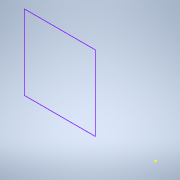
# Autodesk Inventor part: electronics box
Saved by Autodesk Inventor 2022 (Build 260153000, 153)
## iProperties
Created: 2022-02-07
Part Number: electronics box
Material: Generic
Document SubType Name: Modeling
Designer: efred
Density: 1 g/cm^3
Appearance: Default
Author: efred
Autodesk Inventor part; units mm, degrees
ref_plane "YZ Plane" through (0, 0, 0) normal (1, 0, 0) x (0, 1, 0)
ref_plane "XZ Plane" through (0, 0, 0) normal (0, 1, 0) x (-1, 0, 0)
ref_plane "XY Plane" through (0, 0, 0) normal (0, 0, 1) x (1, 0, 0)
sketch "Sketch1" plane through (0, 0, 0) normal (0, 0, 1) x (1, 0, 0)
  line L0 (-184.2713, 193.3742) -> (-404.2713, 193.3742)
  line L1 (-404.2713, 193.3742) -> (-404.2713, -23.6258)
  line L2 (-404.2713, -23.6258) -> (-184.2713, -23.6258)
  line L3 (-184.2713, -23.6258) -> (-184.2713, 193.3742)
  line L4 (-196.3213, 183.3742) -> (-190.7713, 183.3742) projected
  point P0 (0, 0)
  dimension "d2" = 10
  dimension "d3" = 217
  dimension "d4" = 220
  constraints: 8 end point, 2 parallel, 1 horizontal, 1 perpendicular
  measures "d2" distance between parallel lines of L4 L0
  measures "d3" distance of L2.end L0.start
  measures "d4" distance of L1.end L2.end
extrude "Extrusion1" add sketch "Sketch1" against normal blind 10
sketch "Sketch2" plane through (0, 0, -10) normal (0, 0, -1) x (-1, 0, 0)
  line L0 (404.2713, -23.6258) -> (404.2713, 193.3742) projected
  line L1 (404.2713, 193.3742) -> (184.2713, 193.3742) projected
  line L2 (184.2713, 193.3742) -> (184.2713, -23.6258) projected
  line L3 (184.2713, -23.6258) -> (404.2713, -23.6258) projected
  circle A0 centre (400.2713, 80.3742) radius 1.5 projected
  circle A1 centre (363.2713, 80.3742) radius 1.5 projected
  circle A2 centre (400.2713, 93.3742) radius 1.5 projected
  circle A3 centre (363.2713, 93.3742) radius 1.5 projected
  circle A4 centre (363.2713, 130.3742) radius 1.5 projected
  circle A5 centre (400.2713, 130.3742) radius 1.5 projected
  circle A6 centre (400.2713, 143.3742) radius 1.5 projected
  circle A7 centre (400.2713, 180.3742) radius 1.5 projected
  circle A8 centre (363.2713, 180.3742) radius 1.5 projected
  circle A9 centre (363.2713, 143.3742) radius 1.5 projected
  circle A10 centre (320.7713, 167.5022) radius 1.375 projected
  circle A11 centre (320.7713, 109.5022) radius 1.375 projected
  circle A12 centre (271.7713, 109.5022) radius 1.375 projected
  circle A13 centre (271.7713, 167.5022) radius 1.375 projected
  circle A14 centre (244.7713, 128.3904) radius 2 projected
  circle A15 centre (244.7713, 100.8904) radius 2 projected
  circle A16 centre (263.7713, 100.8904) radius 2 projected
  circle A17 centre (263.7713, 128.3904) radius 2 projected
  line L4 (264.4663, 47.3647) -> (264.4663, 46.7297) projected
  arc A18 (264.4663, 46.7297) -> (264.5298, 46.6662) centre (264.5298, 46.7297) ccw projected
  line L5 (264.5298, 46.6662) -> (266.003, 46.6662) projected
  arc A19 (266.0665, 46.6027) -> (266.003, 46.6662) centre (266.003, 46.6027) ccw projected
  line L6 (266.0665, 39.1097) -> (266.0665, 46.6027) projected
  arc A20 (266.003, 39.0462) -> (266.0665, 39.1097) centre (266.003, 39.1097) ccw projected
  line L7 (266.003, 39.0462) -> (264.5298, 39.0462) projected
  arc A21 (264.5298, 39.0462) -> (264.4663, 38.9827) centre (264.5298, 38.9827) ccw projected
  line L8 (264.4663, 38.9827) -> (264.4663, 38.3477) projected
  arc A22 (264.4028, 38.2842) -> (264.4663, 38.3477) centre (264.4028, 38.3477) ccw projected
  line L9 (253.6713, 38.2842) -> (264.4028, 38.2842) projected
  line L10 (253.6713, 35.9982) -> (253.6713, 38.2842) projected
  line L11 (253.6713, 35.9982) -> (255.1953, 34.4742) projected
  line L12 (351.7153, 34.4742) -> (255.1953, 34.4742) projected
  line L13 (351.7153, 34.4742) -> (355.2713, 38.0302) projected
  line L14 (355.2713, 72.6504) -> (355.2713, 38.0302) projected
  line L15 (352.7313, 75.1904) -> (355.2713, 72.6504) projected
  line L16 (352.7313, 86.127) -> (352.7313, 75.1904) projected
  line L17 (350.9679, 87.8904) -> (352.7313, 86.127) projected
  line L18 (255.1953, 87.8904) -> (350.9679, 87.8904) projected
  line L19 (255.1953, 87.8904) -> (253.6713, 86.3664) projected
  line L20 (253.6713, 78.6194) -> (253.6713, 86.3664) projected
  line L21 (260.6817, 78.6194) -> (253.6713, 78.6194) projected
  line L22 (260.6817, 78.6829) -> (260.6817, 78.6194) projected
  line L23 (263.6281, 78.6829) -> (260.6817, 78.6829) projected
  line L24 (263.6281, 66.6179) -> (263.6281, 78.6829) projected
  line L25 (263.6281, 66.6179) -> (260.6817, 66.6179) projected
  line L26 (260.6817, 66.6179) -> (260.6817, 66.6814) projected
  line L27 (253.6713, 66.6814) -> (260.6817, 66.6814) projected
  line L28 (253.6713, 47.4282) -> (253.6713, 66.6814) projected
  line L29 (264.4028, 47.4282) -> (253.6713, 47.4282) projected
  arc A23 (264.4663, 47.3647) -> (264.4028, 47.4282) centre (264.4028, 47.3647) ccw projected
  line L30 (301.2963, 35.8204) -> (301.2963, 38.2698) projected
  line L31 (285.5991, 35.8204) -> (301.2963, 35.8204) projected
  line L32 (285.5991, 38.2698) -> (285.5991, 35.8204) projected
  line L33 (301.2963, 38.2698) -> (285.5991, 38.2698) projected
  line L34 (274.9311, 84.1566) -> (295.6829, 84.1566) projected
  line L35 (274.9311, 86.6204) -> (274.9311, 84.1566) projected
  line L36 (295.6829, 86.6204) -> (274.9311, 86.6204) projected
  line L37 (295.6829, 84.1566) -> (295.6829, 86.6204) projected
  line L38 (326.1883, 38.2842) -> (326.1883, 35.8204) projected
  line L39 (347.0163, 38.2842) -> (326.1883, 38.2842) projected
  line L40 (347.0163, 35.8204) -> (347.0163, 38.2842) projected
  line L41 (326.1883, 35.8204) -> (347.0163, 35.8204) projected
  line L42 (351.2073, 40.3924) -> (351.2073, 86.6712) projected
  line L43 (346.2289, 40.3924) -> (351.2073, 40.3924) projected
  line L44 (346.2289, 86.6712) -> (346.2289, 40.3924) projected
  line L45 (351.2073, 86.6712) -> (346.2289, 86.6712) projected
  line L46 (320.3971, 86.6204) -> (320.3971, 84.1566) projected
  line L47 (341.1489, 86.6204) -> (320.3971, 86.6204) projected
  line L48 (341.1489, 84.1566) -> (341.1489, 86.6204) projected
  line L49 (320.3971, 84.1566) -> (341.1489, 84.1566) projected
  line L50 (297.6641, 84.1566) -> (318.4159, 84.1566) projected
  line L51 (297.6641, 86.6204) -> (297.6641, 84.1566) projected
  line L52 (318.4159, 86.6204) -> (297.6641, 86.6204) projected
  line L53 (318.4159, 84.1566) -> (318.4159, 86.6204) projected
  line L54 (303.4553, 35.8204) -> (324.2833, 35.8204) projected
  line L55 (303.4553, 38.2842) -> (303.4553, 35.8204) projected
  line L56 (324.2833, 38.2842) -> (303.4553, 38.2842) projected
  line L57 (324.2833, 35.8204) -> (324.2833, 38.2842) projected
  line L58 (280.1404, 60.0164) -> (280.1404, 58.6083) projected
  line L59 (282.9054, 60.0164) -> (280.1404, 60.0164) projected
  line L60 (282.9054, 58.6083) -> (282.9054, 60.0164) projected
  line L61 (280.1404, 58.6083) -> (282.9054, 58.6083) projected
  line L62 (260.5311, 55.1409) -> (260.5311, 48.6482) projected
  line L63 (263.8001, 55.1409) -> (260.5311, 55.1409) projected
  line L64 (263.8001, 48.6482) -> (263.8001, 55.1409) projected
  line L65 (260.5311, 48.6482) -> (263.8001, 48.6482) projected
  line L66 (270.6715, 56.9261) -> (270.6715, 54.065) projected
  line L67 (273.4919, 56.9261) -> (270.6715, 56.9261) projected
  line L68 (273.4919, 54.065) -> (273.4919, 56.9261) projected
  line L69 (270.6715, 54.065) -> (273.4919, 54.065) projected
  line L70 (274.4255, 51.6909) -> (274.4255, 50.9604) projected
  line L71 (276.0217, 51.6909) -> (274.4255, 51.6909) projected
  line L72 (276.0217, 50.9604) -> (276.0217, 51.6909) projected
  line L73 (274.4255, 50.9604) -> (276.0217, 50.9604) projected
  line L74 (256.3541, 63.1285) -> (256.3541, 58.6083) projected
  line L75 (259.5172, 63.1285) -> (256.3541, 63.1285) projected
  line L76 (259.5172, 58.6083) -> (259.5172, 63.1285) projected
  line L77 (256.3541, 58.6083) -> (259.5172, 58.6083) projected
  line L78 (291.5916, 41.6564) -> (291.5916, 40.9303) projected
  line L79 (293.1393, 41.6564) -> (291.5916, 41.6564) projected
  line L80 (293.1393, 40.9303) -> (293.1393, 41.6564) projected
  line L81 (291.5916, 40.9303) -> (293.1393, 40.9303) projected
  line L82 (293.7611, 49.5648) -> (293.7611, 48.1079) projected
  line L83 (294.7627, 49.5648) -> (293.7611, 49.5648) projected
  line L84 (294.7627, 48.1079) -> (294.7627, 49.5648) projected
  line L85 (293.7611, 48.1079) -> (294.7627, 48.1079) projected
  line L86 (288.3803, 50.4207) -> (288.3803, 47.161) projected
  line L87 (290.2322, 50.4207) -> (288.3803, 50.4207) projected
  line L88 (290.2322, 47.161) -> (290.2322, 50.4207) projected
  line L89 (288.3803, 47.161) -> (290.2322, 47.161) projected
  line L90 (280.9006, 56.1124) -> (280.9006, 55.3512) projected
  line L91 (282.4644, 56.1124) -> (280.9006, 56.1124) projected
  line L92 (282.4644, 55.3512) -> (282.4644, 56.1124) projected
  line L93 (280.9006, 55.3512) -> (282.4644, 55.3512) projected
  line L94 (264.9561, 63.8625) -> (264.9561, 63.1285) projected
  line L95 (266.426, 63.8625) -> (264.9561, 63.8625) projected
  line L96 (266.426, 63.1285) -> (266.426, 63.8625) projected
  line L97 (264.9561, 63.1285) -> (266.426, 63.1285) projected
  line L98 (271.2991, 63.995) -> (271.2991, 63.1285) projected
  line L99 (272.8749, 63.995) -> (271.2991, 63.995) projected
  line L100 (272.8749, 63.1285) -> (272.8749, 63.995) projected
  line L101 (271.2991, 63.1285) -> (272.8749, 63.1285) projected
  line L102 (277.5304, 63.995) -> (277.5304, 63.1285) projected
  line L103 (279.0938, 63.995) -> (277.5304, 63.995) projected
  line L104 (279.0938, 63.1285) -> (279.0938, 63.995) projected
  line L105 (277.5304, 63.1285) -> (279.0938, 63.1285) projected
  line L106 (280.586, 69.1892) -> (280.586, 67.9164) projected
  line L107 (282.364, 69.1892) -> (280.586, 69.1892) projected
  line L108 (282.364, 67.9164) -> (282.364, 69.1892) projected
  line L109 (280.586, 67.9164) -> (282.364, 67.9164) projected
  line L110 (281.1017, 75.279) -> (281.1017, 72.0231) projected
  line L111 (281.9552, 75.279) -> (281.1017, 75.279) projected
  line L112 (281.9552, 72.0231) -> (281.9552, 75.279) projected
  line L113 (281.1017, 72.0231) -> (281.9552, 72.0231) projected
  line L114 (280.723, 79.124) -> (280.723, 78.3693) projected
  line L115 (282.1593, 79.124) -> (280.723, 79.124) projected
  line L116 (282.1593, 78.3693) -> (282.1593, 79.124) projected
  line L117 (280.723, 78.3693) -> (282.1593, 78.3693) projected
  line L118 (264.8237, 76.8639) -> (264.8237, 76.0914) projected
  line L119 (266.426, 76.8639) -> (264.8237, 76.8639) projected
  line L120 (266.426, 76.0914) -> (266.426, 76.8639) projected
  line L121 (264.8237, 76.0914) -> (266.426, 76.0914) projected
  line L122 (265.1217, 72.9188) -> (265.1217, 69.7454) projected
  line L123 (266.0847, 72.9188) -> (265.1217, 72.9188) projected
  line L124 (266.0847, 69.7454) -> (266.0847, 72.9188) projected
  line L125 (265.1217, 69.7454) -> (266.0847, 69.7454) projected
  line L126 (329.347, 72.0231) -> (329.347, 70.6029) projected
  line L127 (331.1516, 72.0231) -> (329.347, 72.0231) projected
  line L128 (331.1516, 70.6029) -> (331.1516, 72.0231) projected
  line L129 (329.347, 70.6029) -> (331.1516, 70.6029) projected
  line L130 (265.4938, 82.1758) -> (265.4938, 78.9239) projected
  line L131 (267.314, 82.1758) -> (265.4938, 82.1758) projected
  line L132 (267.314, 78.9239) -> (267.314, 82.1758) projected
  line L133 (265.4938, 78.9239) -> (267.314, 78.9239) projected
  arc A24 (268.1885, 62.0274) -> (268.1885, 58.2685) centre (268.5107, 60.148) ccw projected
  line L134 (276.0872, 62.0274) -> (268.1885, 62.0274) projected
  arc A25 (276.0872, 58.2685) -> (276.0872, 62.0274) centre (275.765, 60.148) ccw projected
  line L135 (268.1885, 58.2685) -> (276.0872, 58.2685) projected
  circle A26 centre (278.8902, 43.0749) radius 3.302 projected
  line L136 (321.5903, 61.6809) -> (321.5903, 62.3455) projected
  line L137 (320.5743, 60.6649) -> (321.5903, 61.6809) projected
  line L138 (317.1957, 60.6649) -> (320.5743, 60.6649) projected
  line L139 (316.1797, 61.6809) -> (317.1957, 60.6649) projected
  line L140 (316.1797, 62.3455) -> (316.1797, 61.6809) projected
  line L141 (317.1957, 63.3615) -> (316.1797, 62.3455) projected
  line L142 (320.5743, 63.3615) -> (317.1957, 63.3615) projected
  line L143 (321.5903, 62.3455) -> (320.5743, 63.3615) projected
  line L144 (269.5764, 83.2492) -> (268.916, 83.2492) projected
  line L145 (270.5924, 82.2332) -> (269.5764, 83.2492) projected
  line L146 (270.5924, 78.855) -> (270.5924, 82.2332) projected
  line L147 (269.5764, 77.839) -> (270.5924, 78.855) projected
  line L148 (268.916, 77.839) -> (269.5764, 77.839) projected
  line L149 (267.9, 78.855) -> (268.916, 77.839) projected
  line L150 (267.9, 82.2332) -> (267.9, 78.855) projected
  line L151 (268.916, 83.2492) -> (267.9, 82.2332) projected
  line L152 (274.504, 83.2492) -> (273.488, 82.2332) projected
  line L153 (275.1644, 83.2492) -> (274.504, 83.2492) projected
  line L154 (276.1804, 82.2332) -> (275.1644, 83.2492) projected
  line L155 (276.1804, 78.855) -> (276.1804, 82.2332) projected
  line L156 (275.1644, 77.839) -> (276.1804, 78.855) projected
  line L157 (274.504, 77.839) -> (275.1644, 77.839) projected
  line L158 (273.488, 78.855) -> (274.504, 77.839) projected
  line L159 (273.488, 82.2332) -> (273.488, 78.855) projected
  circle A27 centre (267.7937, 85.3504) radius 1.5621 projected
  circle A28 centre (267.7937, 37.0142) radius 1.5621 projected
  circle A29 centre (350.4199, 37.0142) radius 1.5621 projected
  circle A30 centre (319.4192, 41.8927) radius 1.5621 projected
  circle A31 centre (319.4192, 69.9089) radius 1.3153 projected
  circle A32 centre (342.9269, 85.3504) radius 1.5621 projected
  line L160 (271.71, 83.2492) -> (270.694, 82.2332) projected
  line L161 (272.3704, 83.2492) -> (271.71, 83.2492) projected
  line L162 (273.3864, 82.2332) -> (272.3704, 83.2492) projected
  line L163 (273.3864, 78.855) -> (273.3864, 82.2332) projected
  line L164 (272.3704, 77.839) -> (273.3864, 78.855) projected
  line L165 (271.71, 77.839) -> (272.3704, 77.839) projected
  line L166 (270.694, 78.855) -> (271.71, 77.839) projected
  line L167 (270.694, 82.2332) -> (270.694, 78.855) projected
  line L168 (321.5903, 58.8869) -> (321.5903, 59.5515) projected
  line L169 (320.5743, 57.8709) -> (321.5903, 58.8869) projected
  line L170 (317.1957, 57.8709) -> (320.5743, 57.8709) projected
  line L171 (316.1797, 58.8869) -> (317.1957, 57.8709) projected
  line L172 (316.1797, 59.5515) -> (316.1797, 58.8869) projected
  line L173 (317.1957, 60.5675) -> (316.1797, 59.5515) projected
  line L174 (320.5743, 60.5675) -> (317.1957, 60.5675) projected
  line L175 (321.5903, 59.5515) -> (320.5743, 60.5675) projected
  line L176 (321.5903, 64.4749) -> (321.5903, 65.1395) projected
  line L177 (320.5743, 63.4589) -> (321.5903, 64.4749) projected
  line L178 (317.1957, 63.4589) -> (320.5743, 63.4589) projected
  line L179 (316.1797, 64.4749) -> (317.1957, 63.4589) projected
  line L180 (316.1797, 65.1395) -> (316.1797, 64.4749) projected
  line L181 (317.1957, 66.1555) -> (316.1797, 65.1395) projected
  line L182 (320.5743, 66.1555) -> (317.1957, 66.1555) projected
  line L183 (321.5903, 65.1395) -> (320.5743, 66.1555) projected
  circle A33 centre (271.7013, 43.0749) radius 3.302 projected
  line L184 (324.9856, 65.2513) -> (324.9856, 58.9724) projected
  line L185 (331.4465, 65.2513) -> (324.9856, 65.2513) projected
  line L186 (331.4465, 58.9724) -> (331.4465, 65.2513) projected
  line L187 (324.9856, 58.9724) -> (331.4465, 58.9724) projected
  line L188 (334.0973, 72.9188) -> (334.0973, 69.5148) projected
  line L189 (335.3446, 72.9188) -> (334.0973, 72.9188) projected
  line L190 (335.3446, 69.5148) -> (335.3446, 72.9188) projected
  line L191 (334.0973, 69.5148) -> (335.3446, 69.5148) projected
  line L192 (264.8237, 69.0398) -> (264.8237, 68.1038) projected
  line L193 (266.426, 69.0398) -> (264.8237, 69.0398) projected
  line L194 (266.426, 68.1038) -> (266.426, 69.0398) projected
  line L195 (264.8237, 68.1038) -> (266.426, 68.1038) projected
  line L196 (264.8237, 74.5464) -> (264.8237, 73.651) projected
  line L197 (266.426, 74.5464) -> (264.8237, 74.5464) projected
  line L198 (266.426, 73.651) -> (266.426, 74.5464) projected
  line L199 (264.8237, 73.651) -> (266.426, 73.651) projected
  line L200 (260.7973, 80.0134) -> (260.7973, 78.9239) projected
  line L201 (262.7392, 80.0134) -> (260.7973, 80.0134) projected
  line L202 (262.7392, 78.9239) -> (262.7392, 80.0134) projected
  line L203 (260.7973, 78.9239) -> (262.7392, 78.9239) projected
  line L204 (280.586, 77.0683) -> (280.586, 75.8363) projected
  line L205 (282.364, 77.0683) -> (280.586, 77.0683) projected
  line L206 (282.364, 75.8363) -> (282.364, 77.0683) projected
  line L207 (280.586, 75.8363) -> (282.364, 75.8363) projected
  line L208 (280.586, 71.5023) -> (280.586, 70.2429) projected
  line L209 (282.364, 71.5023) -> (280.586, 71.5023) projected
  line L210 (282.364, 70.2429) -> (282.364, 71.5023) projected
  line L211 (280.586, 70.2429) -> (282.364, 70.2429) projected
  line L212 (281.1017, 66.9428) -> (281.1017, 63.7241) projected
  line L213 (282.1593, 66.9428) -> (281.1017, 66.9428) projected
  line L214 (282.1593, 63.7241) -> (282.1593, 66.9428) projected
  line L215 (281.1017, 63.7241) -> (282.1593, 63.7241) projected
  line L216 (274.4255, 63.995) -> (274.4255, 63.1285) projected
  line L217 (275.9057, 63.995) -> (274.4255, 63.995) projected
  line L218 (275.9057, 63.1285) -> (275.9057, 63.995) projected
  line L219 (274.4255, 63.1285) -> (275.9057, 63.1285) projected
  line L220 (268.0843, 63.8625) -> (268.0843, 63.1285) projected
  line L221 (269.6173, 63.8625) -> (268.0843, 63.8625) projected
  line L222 (269.6173, 63.1285) -> (269.6173, 63.8625) projected
  line L223 (268.0843, 63.1285) -> (269.6173, 63.1285) projected
  line L224 (264.8237, 65.4913) -> (264.8237, 64.816) projected
  line L225 (266.426, 65.4913) -> (264.8237, 65.4913) projected
  line L226 (266.426, 64.816) -> (266.426, 65.4913) projected
  line L227 (264.8237, 64.816) -> (266.426, 64.816) projected
  line L228 (280.8086, 52.8068) -> (280.8086, 52.0587) projected
  line L229 (282.364, 52.8068) -> (280.8086, 52.8068) projected
  line L230 (282.364, 52.0587) -> (282.364, 52.8068) projected
  line L231 (280.8086, 52.0587) -> (282.364, 52.0587) projected
  line L232 (291.4666, 50.4207) -> (291.4666, 47.161) projected
  line L233 (292.7414, 50.4207) -> (291.4666, 50.4207) projected
  line L234 (292.7414, 47.161) -> (292.7414, 50.4207) projected
  line L235 (291.4666, 47.161) -> (292.7414, 47.161) projected
  line L236 (286.7319, 50.0382) -> (286.7319, 47.9076) projected
  line L237 (287.6971, 50.0382) -> (286.7319, 50.0382) projected
  line L238 (287.6971, 47.9076) -> (287.6971, 50.0382) projected
  line L239 (286.7319, 47.9076) -> (287.6971, 47.9076) projected
  line L240 (262.1656, 61.3744) -> (262.1656, 58.6083) projected
  line L241 (263.3129, 61.3744) -> (262.1656, 61.3744) projected
  line L242 (263.3129, 58.6083) -> (263.3129, 61.3744) projected
  line L243 (262.1656, 58.6083) -> (263.3129, 58.6083) projected
  line L244 (267.6886, 52.5228) -> (267.6886, 50.9604) projected
  line L245 (268.48, 52.5228) -> (267.6886, 52.5228) projected
  line L246 (268.48, 50.9604) -> (268.48, 52.5228) projected
  line L247 (267.6886, 50.9604) -> (268.48, 50.9604) projected
  line L248 (271.6658, 52.259) -> (271.6658, 49.053) projected
  line L249 (272.6195, 52.259) -> (271.6658, 52.259) projected
  line L250 (272.6195, 49.053) -> (272.6195, 52.259) projected
  line L251 (271.6658, 49.053) -> (272.6195, 49.053) projected
  line L252 (273.2984, 38.1367) -> (273.2984, 35.6899) projected
  line L253 (277.3334, 38.1367) -> (273.2984, 38.1367) projected
  line L254 (277.3334, 35.6899) -> (277.3334, 38.1367) projected
  line L255 (273.2984, 35.6899) -> (277.3334, 35.6899) projected
  line L256 (270.9621, 71.5023) -> (270.9621, 66.5772) projected
  line L257 (276.0217, 71.5023) -> (270.9621, 71.5023) projected
  line L258 (276.0217, 66.5772) -> (276.0217, 71.5023) projected
  line L259 (270.9621, 66.5772) -> (276.0217, 66.5772) projected
  line L260 (297.5109, 69.7454) -> (297.5109, 55.5474) projected
  line L261 (311.5444, 69.7454) -> (297.5109, 69.7454) projected
  line L262 (311.5444, 55.5474) -> (311.5444, 69.7454) projected
  line L263 (297.5109, 55.5474) -> (311.5444, 55.5474) projected
  arc A34 (196.3213, 78.3742) -> (200.8213, 78.3742) centre (198.5713, 78.3742) ccw projected
  arc A35 (200.8213, -8.6258) -> (196.3213, -8.6258) centre (198.5713, -8.6258) ccw projected
  line L264 (209.2713, 93.8742) -> (190.7713, 93.8742) projected
  line L265 (190.7713, 86.3742) -> (190.7713, 93.8742) projected
  line L266 (196.3213, 86.3742) -> (190.7713, 86.3742) projected
  line L267 (196.3213, 86.3742) -> (196.3213, 91.3742) projected
  arc A36 (200.8213, 91.3742) -> (196.3213, 91.3742) centre (198.5713, 91.3742) ccw projected
  line L268 (200.8213, 91.3742) -> (200.8213, 86.3742) projected
  line L269 (210.3213, 86.3742) -> (200.8213, 86.3742) projected
  line L270 (210.3213, 86.3742) -> (210.3213, 183.3742) projected
  line L271 (210.3213, 183.3742) -> (200.8213, 183.3742) projected
  line L272 (200.8213, 178.3742) -> (200.8213, 183.3742) projected
  arc A37 (196.3213, 178.3742) -> (200.8213, 178.3742) centre (198.5713, 178.3742) ccw projected
  line L273 (196.3213, 183.3742) -> (196.3213, 178.3742) projected
  line L274 (196.3213, 183.3742) -> (190.7713, 183.3742) projected
  line L275 (190.7713, 175.8742) -> (190.7713, 183.3742) projected
  line L276 (190.7713, 175.8742) -> (209.2713, 175.8742) projected
  arc A38 (210.2713, 174.8742) -> (209.2713, 175.8742) centre (209.2713, 174.8742) ccw projected
  line L277 (210.2713, 174.8742) -> (210.2713, 94.8742) projected
  arc A39 (209.2713, 93.8742) -> (210.2713, 94.8742) centre (209.2713, 94.8742) ccw projected
  circle A40 centre (198.5713, -8.6258) radius 2
  circle A41 centre (198.5713, 78.3742) radius 2
  circle A42 centre (198.5713, 91.3742) radius 2
  circle A43 centre (198.5713, 178.3742) radius 2
  circle A44 centre (363.2713, 43.3742) radius 1.5 projected
  circle A45 centre (400.2713, 43.3742) radius 1.5 projected
  point P0 (0, 0)
  dimension "d5" = 4
  dimension "d6" = 4
  dimension "d7" = 4
  dimension "d8" = 4
  constraints: 4 centre point, 4 coincident
  measures "d5" diameter of A40
  measures "d6" diameter of A41
  measures "d7" diameter of A42
  measures "d8" diameter of A43
extrude "Extrusion2" cut sketch "Sketch2" against normal through all contours A0 | A1 | A2 | A3 | A4 | A5 | A6 | A7 | A8 | A9 | A10 | A11 | A12 | A13 | A14 | A15 | A16 | A17 | A27 | A28 | A29 | A30 | A31 | A32 | A40 | A41 | A42 | A43 | A44 | A45
sketch "Sketch3" plane through (0, 0, 0) normal (0, 0, 1) x (1, 0, 0)
  line L0 (-184.2713, 193.3742) -> (-404.2713, 193.3742) projected
  line L1 (-404.2713, 193.3742) -> (-184.2713, 193.3742)
  line L2 (-184.2713, 193.3742) -> (-184.2713, 198.3742)
  line L3 (-184.2713, 198.3742) -> (-404.2713, 198.3742)
  line L4 (-404.2713, 198.3742) -> (-404.2713, 193.3742)
  line L5 (-404.2713, -23.6258) -> (-404.2713, 193.3742) projected
  line L6 (-404.2713, -23.6258) -> (-184.2713, -23.6258)
  line L7 (-184.2713, -23.6258) -> (-184.2713, -28.6258)
  line L8 (-184.2713, -28.6258) -> (-404.2713, -28.6258)
  line L9 (-404.2713, -28.6258) -> (-404.2713, -23.6258)
  line L10 (-184.2713, -23.6258) -> (-184.2713, 193.3742) projected
  line L11 (-324.2713, 193.3742) -> (-268.2713, 193.3742)
  line L12 (-268.2713, 193.3742) -> (-268.2713, 198.3742)
  line L13 (-268.2713, 198.3742) -> (-324.2713, 198.3742)
  line L14 (-324.2713, 198.3742) -> (-324.2713, 193.3742)
  line L15 (-324.2713, 187.9264) -> (-324.2713, 109.0022) projected
  line L16 (-268.2713, 109.0022) -> (-268.2713, 187.9264) projected
  point P0 (0, 0)
  dimension "d11" = 5
  dimension "d12" = 5
  constraints: 24 end point, 6 parallel, 3 collinear, 3 horizontal, 3 perpendicular, 2 point on line
  measures "d11" distance between parallel lines of L0 L3
  measures "d12" distance between parallel lines of L6 L8
extrude "Extrusion3" add sketch "Sketch3" against normal blind 100 contours L0 L12 L3 L2 | L7 L8 L9 L6 | L0 L4 L3 L14
fillet "Fillet1" radius 5 2 edges at (-324.2713, 193.3742, -5) (-268.2713, 193.3742, -5)
body "Solid1"
